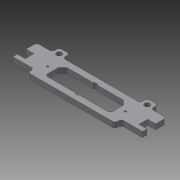
# Autodesk Inventor part: camera_mount_v1
Saved by Autodesk Inventor 2016 (Build 200138000, 138)
## iProperties
Created: 2015-06-17
Part Number: camera_mount_v1
Material: Generic
Document SubType Name: Modeling
Designer: Robert Allen Fett
Density: 1 g/cm^3
Appearance: Default
Author: Robert Allen Fett
Autodesk Inventor part; units mm, degrees
ref_plane "YZ Plane" through (0, 0, 0) normal (1, 0, 0) x (0, 1, 0)
ref_plane "XZ Plane" through (0, 0, 0) normal (0, 1, 0) x (-1, 0, 0)
ref_plane "XY Plane" through (0, 0, 0) normal (0, 0, 1) x (1, 0, 0)
sketch "Sketch1" plane through (0, 0, 0) normal (0, 0, 1) x (1, 0, 0)
  line L0 (-73.5, -17) -> (73.5, -17)
  line L1 (73.5, -17) -> (73.5, 17)
  line L2 (73.5, 17) -> (-73.5, 17)
  line L3 (-73.5, 17) -> (-73.5, -17)
  line L4 (-73.5, -17) -> (73.5, 17) construction
  line L5 (73.5, -17) -> (-73.5, 17) construction
  point P0 (0, 0)
  dimension "d0" = 147
  dimension "d1" = 34
  constraints: 12 end point, 2 midpoint, 2 parallel, 1 horizontal, 1 perpendicular
  measures "d0" distance of L2.end L1.end
  measures "d1" distance of L2.end L0.start
extrude "Extrusion1" add sketch "Sketch1" along normal blind 6
sketch "Sketch2" plane through (0, 0, 6) normal (0, 0, 1) x (1, 0, 0)
  line L0 (-37, -10) -> (37, -10)
  line L1 (37, -10) -> (37, 10)
  line L2 (37, 10) -> (-37, 10)
  line L3 (-37, 10) -> (-37, -10)
  line L4 (-37, -10) -> (37, 10) construction
  line L5 (37, -10) -> (-37, 10) construction
  point P0 (0, 0)
  dimension "d4" = 74
  dimension "d5" = 20
  constraints: 12 end point, 2 midpoint, 2 parallel, 1 horizontal, 1 perpendicular
  measures "d4" distance of L2.end L1.end
  measures "d5" distance of L1.end L0.end
extrude "Extrusion2" cut sketch "Sketch2" against normal blind 6
sketch "Sketch3" plane through (0, 0, 6) normal (0, 0, 1) x (1, 0, 0)
  circle A0 centre (0, 9) radius 2.5
  circle A1 centre (0, -9) radius 2.5
  point P0 (0, 0)
  dimension "d8" = 5
  dimension "d10" = 9
  dimension "d11" = 5
  dimension "d12" = 9
  constraints: 2 centre point, 2 vertical alignment
  measures "d8" diameter of A0
  measures "d10" distance of point (0, 0) A0.centre
  measures "d11" diameter of A1
  measures "d12" distance of A1.centre point (0, 0)
extrude "Extrusion3" cut sketch "Sketch3" against normal blind 6
sketch "Sketch4" plane through (0, 0, 6) normal (0, 0, 1) x (1, 0, 0)
  line L0 (73.5, 17) -> (-73.5, 17) projected
  circle A0 centre (-50, 19) radius 3
  line L1 (-56, 13) -> (-44, 13)
  line L2 (-44, 13) -> (-44, 25)
  line L3 (-44, 25) -> (-56, 25)
  line L4 (-56, 25) -> (-56, 13)
  line L5 (-56, 13) -> (-44, 25) construction
  line L6 (-44, 13) -> (-56, 25) construction
  point P0 (0, 0)
  dimension "d15" = 6
  dimension "d16" = 12
  dimension "d17" = 12
  dimension "d18" = 50
  dimension "d19" = 2
  constraints: 12 end point, 2 midpoint, 2 parallel, 1 centre point, 1 horizontal, 1 perpendicular
  measures "d15" diameter of A0
  measures "d16" distance of L3.end L2.end
  measures "d17" distance of L2.end L1.end
  measures "d18" horizontal distance of point (0, 0) A0.centre
  measures "d19" distance from line of L0 A0.centre
extrude "Extrusion4" add sketch "Sketch4" against normal blind 6 contours L2 L1 L4 L0 A0 | L0 A0 L4 L3 L2
sketch "Sketch5" plane through (0, 0, 6) normal (0, 0, 1) x (1, 0, 0)
  line L0 (-73.5, 17) -> (-73.5, -17) projected
  line L1 (-37, -10) -> (-37, 10) projected
  line L2 (-73.5, 5) -> (-64.5, 5)
  line L3 (-64.5, 5) -> (-64.5, -5)
  line L4 (-64.5, -5) -> (-73.5, -5)
  line L5 (-73.5, -5) -> (-73.5, 5)
  point P0 (0, 0)
  point P1 (-73.5, 0)
  point P2 (-37, 0)
  dimension "d22" = 9
  dimension "d23" = 10
  constraints: 8 end point, 2 midpoint, 2 parallel, 1 horizontal, 1 horizontal alignment, 1 perpendicular, 1 point on line
  measures "d22" distance of L3.end L4.end
  measures "d23" distance of L2.end L3.end
extrude "Extrusion5" cut sketch "Sketch5" against normal blind 6
sketch "Sketch6" plane through (0, 0, 6) normal (0, 0, 1) x (1, 0, 0)
  line L0 (-73.5, -17) -> (-49.5, -17)
  line L1 (-49.5, -17) -> (-49.5, -10)
  line L2 (-49.5, -10) -> (-73.5, -10)
  line L3 (-73.5, -10) -> (-73.5, -17)
  point P0 (0, 0)
  dimension "d26" = 24
  dimension "d28" = 7
  constraints: 8 end point, 2 parallel, 1 horizontal, 1 perpendicular
  measures "d26" distance of L1.end L2.end
  measures "d28" distance of L0.end L1.end
extrude "Extrusion6" cut sketch "Sketch6" against normal blind 6
sketch "Sketch7" plane through (0, 0, 6) normal (0, 0, 1) x (1, 0, 0)
  line L0 (-37, -10) -> (-37, 10) projected
  circle A0 centre (-44.1, 0) radius 1.125
  point P0 (0, 0)
  point P1 (-37, 0)
  dimension "d31" = 2.25
  dimension "d32" = 44.1
  constraints: 1 centre point, 1 horizontal alignment, 1 midpoint
  measures "d31" diameter of A0
  measures "d32" distance of point (0, 0) A0.centre
extrude "Extrusion7" cut sketch "Sketch7" against normal blind 6
mirror "Mirror1" about plane through (0, 0, 0) normal (1, 0, 0) of "Extrusion4", "Extrusion5", "Extrusion6", "Extrusion7"
chamfer "Chamfer3" distance 5 angle 45 2 edges at (-37, 10, 3) (37, 10, 3)
chamfer "Chamfer4" distance 2 angle 45 4 edges at (-37, -10, 3) (-49.5, -10, 3) (37, -10, 3) (49.5, -10, 3)
fillet "Fillet2" radius 3 12 edges at (-73.5, 17, 3) (-56, 17, 3) (-56, 25, 3) (-44, 25, 3) (-44, 17, 3) (-49.5, -17, 3) (49.5, -17, 3) (73.5, 17, 3) (56, 17, 3) (56, 25, 3) (44, 25, 3) (44, 17, 3)
sketch "Sketch8" plane through (0, 0, 6) normal (0, 0, 1) x (1, 0, 0)
  circle A0 centre (50, 19) radius 3
  circle A1 centre (-50, 19) radius 3
  arc A2 (-47.7639, 17) -> (-52.2361, 17) centre (-50, 19) ccw projected
  arc A3 (52.2361, 17) -> (47.7639, 17) centre (50, 19) ccw projected
  point P0 (0, 0)
  constraints: 4 concentric, 2 centre point
extrude "Extrusion8" cut sketch "Sketch8" against normal through all
body "Solid1"
